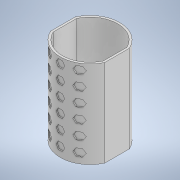
# Autodesk Inventor part: CanSat
Saved by Autodesk Inventor 2022 (Build 260153000, 153)
## iProperties
Created: 2022-01-26
Part Number: CanSat
Material: Generic
Document SubType Name: Modeling
Designer: jtgar
Density: 1 g/cm^3
Appearance: Default
Author: jtgar
Autodesk Inventor part; units mm, degrees
ref_plane "YZ Plane" through (0, 0, 0) normal (1, 0, 0) x (0, 1, 0)
ref_plane "XZ Plane" through (0, 0, 0) normal (0, 1, 0) x (-1, 0, 0)
ref_plane "XY Plane" through (0, 0, 0) normal (0, 0, 1) x (1, 0, 0)
sketch "Sketch1" plane through (0, 0, 0) normal (0, 1, 0) x (-1, 0, 0)
  circle A0 centre (0, 0) radius 28.5
  dimension "d0" = 57
  constraints: 1 centre point, 1 coincident
  measures "d0" diameter of A0
extrude "Extrusion1" add sketch "Sketch1" along normal blind 2.5
sketch "Sketch2" plane through (0, 2.5, 0) normal (0, 1, 0) x (1, 0, 0)
  circle A0 centre (0, 0) radius 27.5
  circle A1 centre (0, 0) radius 28.5
  dimension "d3" = 55
  dimension "d4" = 57
  constraints: 2 centre point, 2 coincident
  measures "d3" diameter of A0
  measures "d4" diameter of A1
sketch "Sketch3" plane through (0, 0, 0) normal (0, 0, 1) x (1, 0, 0)
  line L0 (-4.0696, 9.3373) -> (-2.0348, 12.8616)
  line L1 (-2.0348, 12.8616) -> (2.0348, 12.8616)
  line L2 (2.0348, 12.8616) -> (4.0696, 9.3373)
  line L3 (4.0696, 9.3373) -> (2.0348, 5.8129)
  line L4 (2.0348, 5.8129) -> (-2.0348, 5.8129)
  line L5 (-2.0348, 5.8129) -> (-4.0696, 9.3373)
  line L6 (4.0696, 9.3373) -> (2.0348, 12.8616)
  line L7 (2.0348, 12.8616) -> (-2.0348, 12.8616)
  line L8 (-2.0348, 12.8616) -> (-4.0696, 9.3373)
  line L9 (-4.0696, 9.3373) -> (-2.0348, 5.8129)
  line L10 (-2.0348, 5.8129) -> (2.0348, 5.8129)
  line L11 (2.0348, 5.8129) -> (4.0696, 9.3373)
  line L12 (4.0696, 9.3373) -> (2.0348, 12.8616)
  line L13 (2.0348, 12.8616) -> (-2.0348, 12.8616)
  line L14 (-2.0348, 12.8616) -> (-4.0696, 9.3373)
  line L15 (-4.0696, 9.3373) -> (-2.0348, 5.8129)
  line L16 (-2.0348, 5.8129) -> (2.0348, 5.8129)
  line L17 (2.0348, 5.8129) -> (4.0696, 9.3373)
  line L18 (-4.0696, 9.3373) -> (-2.0348, 12.8616)
  line L19 (-2.0348, 12.8616) -> (2.0348, 12.8616)
  line L20 (2.0348, 12.8616) -> (4.0696, 9.3373)
  line L21 (4.0696, 9.3373) -> (2.0348, 5.8129)
  line L22 (2.0348, 5.8129) -> (-2.0348, 5.8129)
  line L23 (-2.0348, 5.8129) -> (-4.0696, 9.3373)
  line L24 (28.5, 2.5) -> (-28.5, 2.5) projected
  line L25 (10.1843, 9.3373) -> (12.2172, 12.8582)
  line L26 (12.2172, 12.8582) -> (16.2828, 12.8582)
  line L27 (16.2828, 12.8582) -> (18.3157, 9.3373)
  line L28 (18.3157, 9.3373) -> (16.2828, 5.8163)
  line L29 (16.2828, 5.8163) -> (12.2172, 5.8163)
  line L30 (12.2172, 5.8163) -> (10.1843, 9.3373)
  line L31 (-18.3152, 9.3373) -> (-16.2826, 12.8579)
  line L32 (-16.2826, 12.8579) -> (-12.2174, 12.8579)
  line L33 (-12.2174, 12.8579) -> (-10.1848, 9.3373)
  line L34 (-10.1848, 9.3373) -> (-12.2174, 5.8166)
  line L35 (-12.2174, 5.8166) -> (-16.2826, 5.8166)
  line L36 (-16.2826, 5.8166) -> (-18.3152, 9.3373)
  line L37 (-4.0696, 23.012) -> (-2.0348, 19.4877)
  line L38 (-2.0348, 19.4877) -> (2.0348, 19.4877)
  line L39 (2.0348, 19.4877) -> (4.0696, 23.012)
  line L40 (4.0696, 23.012) -> (2.0348, 26.5364)
  line L41 (2.0348, 26.5364) -> (-2.0348, 26.5364)
  line L42 (-2.0348, 26.5364) -> (-4.0696, 23.012)
  line L43 (4.0696, 23.012) -> (2.0348, 19.4877)
  line L44 (2.0348, 19.4877) -> (-2.0348, 19.4877)
  line L45 (-2.0348, 19.4877) -> (-4.0696, 23.012)
  line L46 (-4.0696, 23.012) -> (-2.0348, 26.5364)
  line L47 (-2.0348, 26.5364) -> (2.0348, 26.5364)
  line L48 (2.0348, 26.5364) -> (4.0696, 23.012)
  line L49 (4.0696, 23.012) -> (2.0348, 19.4877)
  line L50 (2.0348, 19.4877) -> (-2.0348, 19.4877)
  line L51 (-2.0348, 19.4877) -> (-4.0696, 23.012)
  line L52 (-4.0696, 23.012) -> (-2.0348, 26.5364)
  line L53 (-2.0348, 26.5364) -> (2.0348, 26.5364)
  line L54 (2.0348, 26.5364) -> (4.0696, 23.012)
  line L55 (-4.0696, 23.012) -> (-2.0348, 19.4877)
  line L56 (-2.0348, 19.4877) -> (2.0348, 19.4877)
  line L57 (2.0348, 19.4877) -> (4.0696, 23.012)
  line L58 (4.0696, 23.012) -> (2.0348, 26.5364)
  line L59 (2.0348, 26.5364) -> (-2.0348, 26.5364)
  line L60 (-2.0348, 26.5364) -> (-4.0696, 23.012)
  line L61 (10.1843, 23.012) -> (12.2172, 19.491)
  line L62 (12.2172, 19.491) -> (16.2828, 19.491)
  line L63 (16.2828, 19.491) -> (18.3157, 23.012)
  line L64 (18.3157, 23.012) -> (16.2828, 26.533)
  line L65 (16.2828, 26.533) -> (12.2172, 26.533)
  line L66 (12.2172, 26.533) -> (10.1843, 23.012)
  line L67 (-18.3152, 23.012) -> (-16.2826, 19.4914)
  line L68 (-16.2826, 19.4914) -> (-12.2174, 19.4914)
  line L69 (-12.2174, 19.4914) -> (-10.1848, 23.012)
  line L70 (-10.1848, 23.012) -> (-12.2174, 26.5326)
  line L71 (-12.2174, 26.5326) -> (-16.2826, 26.5326)
  line L72 (-16.2826, 26.5326) -> (-18.3152, 23.012)
  line L73 (-4.0696, 50.362) -> (-2.0348, 46.8377)
  line L74 (-2.0348, 46.8377) -> (2.0348, 46.8377)
  line L75 (2.0348, 46.8377) -> (4.0696, 50.362)
  line L76 (4.0696, 50.362) -> (2.0348, 53.8864)
  line L77 (2.0348, 53.8864) -> (-2.0348, 53.8864)
  line L78 (-2.0348, 53.8864) -> (-4.0696, 50.362)
  line L79 (4.0696, 50.362) -> (2.0348, 46.8377)
  line L80 (2.0348, 46.8377) -> (-2.0348, 46.8377)
  line L81 (-2.0348, 46.8377) -> (-4.0696, 50.362)
  line L82 (-4.0696, 50.362) -> (-2.0348, 53.8864)
  line L83 (-2.0348, 53.8864) -> (2.0348, 53.8864)
  line L84 (2.0348, 53.8864) -> (4.0696, 50.362)
  line L85 (4.0696, 50.362) -> (2.0348, 46.8377)
  line L86 (2.0348, 46.8377) -> (-2.0348, 46.8377)
  line L87 (-2.0348, 46.8377) -> (-4.0696, 50.362)
  line L88 (-4.0696, 50.362) -> (-2.0348, 53.8864)
  line L89 (-2.0348, 53.8864) -> (2.0348, 53.8864)
  line L90 (2.0348, 53.8864) -> (4.0696, 50.362)
  line L91 (-4.0696, 50.362) -> (-2.0348, 46.8377)
  line L92 (-2.0348, 46.8377) -> (2.0348, 46.8377)
  line L93 (2.0348, 46.8377) -> (4.0696, 50.362)
  line L94 (4.0696, 50.362) -> (2.0348, 53.8864)
  line L95 (2.0348, 53.8864) -> (-2.0348, 53.8864)
  line L96 (-2.0348, 53.8864) -> (-4.0696, 50.362)
  line L97 (10.1843, 50.362) -> (12.2172, 46.841)
  line L98 (12.2172, 46.841) -> (16.2828, 46.841)
  line L99 (16.2828, 46.841) -> (18.3157, 50.362)
  line L100 (18.3157, 50.362) -> (16.2828, 53.883)
  line L101 (16.2828, 53.883) -> (12.2172, 53.883)
  line L102 (12.2172, 53.883) -> (10.1843, 50.362)
  line L103 (-18.3152, 50.362) -> (-16.2826, 46.8414)
  line L104 (-16.2826, 46.8414) -> (-12.2174, 46.8414)
  line L105 (-12.2174, 46.8414) -> (-10.1848, 50.362)
  line L106 (-10.1848, 50.362) -> (-12.2174, 53.8826)
  line L107 (-12.2174, 53.8826) -> (-16.2826, 53.8826)
  line L108 (-16.2826, 53.8826) -> (-18.3152, 50.362)
  line L109 (-2.0348, 33.1629) -> (2.0348, 33.1629)
  line L110 (-2.0348, 33.1629) -> (2.0348, 33.1629)
  line L111 (2.0348, 33.1629) -> (-2.0348, 33.1629)
  line L112 (2.0348, 33.1629) -> (-2.0348, 33.1629)
  line L113 (4.0696, 36.6873) -> (2.0348, 33.1629)
  line L114 (4.0696, 36.6873) -> (2.0348, 33.1629)
  line L115 (2.0348, 33.1629) -> (4.0696, 36.6873)
  line L116 (2.0348, 33.1629) -> (4.0696, 36.6873)
  line L117 (2.0348, 40.2116) -> (4.0696, 36.6873)
  line L118 (4.0696, 36.6873) -> (2.0348, 40.2116)
  line L119 (4.0696, 36.6873) -> (2.0348, 40.2116)
  line L120 (2.0348, 40.2116) -> (4.0696, 36.6873)
  line L121 (2.0348, 40.2116) -> (-2.0348, 40.2116)
  line L122 (2.0348, 40.2116) -> (-2.0348, 40.2116)
  line L123 (-2.0348, 40.2116) -> (2.0348, 40.2116)
  line L124 (-2.0348, 40.2116) -> (2.0348, 40.2116)
  line L125 (10.1843, 36.6873) -> (12.2172, 40.2082)
  line L126 (12.2172, 33.1663) -> (10.1843, 36.6873)
  line L127 (12.2172, 40.2082) -> (16.2828, 40.2082)
  line L128 (16.2828, 33.1663) -> (12.2172, 33.1663)
  line L129 (18.3157, 36.6873) -> (16.2828, 33.1663)
  line L130 (16.2828, 40.2082) -> (18.3157, 36.6873)
  line L131 (-4.0696, 36.6873) -> (-2.0348, 40.2116)
  line L132 (-2.0348, 33.1629) -> (-4.0696, 36.6873)
  line L133 (-2.0348, 40.2116) -> (-4.0696, 36.6873)
  line L134 (-4.0696, 36.6873) -> (-2.0348, 33.1629)
  line L135 (-2.0348, 40.2116) -> (-4.0696, 36.6873)
  line L136 (-4.0696, 36.6873) -> (-2.0348, 33.1629)
  line L137 (-4.0696, 36.6873) -> (-2.0348, 40.2116)
  line L138 (-2.0348, 33.1629) -> (-4.0696, 36.6873)
  line L139 (-12.2174, 40.2079) -> (-10.1848, 36.6873)
  line L140 (-16.2826, 40.2079) -> (-12.2174, 40.2079)
  line L141 (-12.2174, 33.1666) -> (-16.2826, 33.1666)
  line L142 (-18.3152, 36.6873) -> (-16.2826, 40.2079)
  line L143 (-16.2826, 33.1666) -> (-18.3152, 36.6873)
  line L144 (-10.1848, 36.6873) -> (-12.2174, 33.1666)
  line L145 (-4.0696, 105.0625) -> (-2.0348, 101.5381)
  line L146 (-2.0348, 101.5381) -> (2.0348, 101.5381)
  line L147 (2.0348, 101.5381) -> (4.0696, 105.0625)
  line L148 (4.0696, 105.0625) -> (2.0348, 108.5868)
  line L149 (2.0348, 108.5868) -> (-2.0348, 108.5868)
  line L150 (-2.0348, 108.5868) -> (-4.0696, 105.0625)
  line L151 (4.0696, 105.0625) -> (2.0348, 101.5381)
  line L152 (2.0348, 101.5381) -> (-2.0348, 101.5381)
  line L153 (-2.0348, 101.5381) -> (-4.0696, 105.0625)
  line L154 (-4.0696, 105.0625) -> (-2.0348, 108.5868)
  line L155 (-2.0348, 108.5868) -> (2.0348, 108.5868)
  line L156 (2.0348, 108.5868) -> (4.0696, 105.0625)
  line L157 (4.0696, 105.0625) -> (2.0348, 101.5381)
  line L158 (2.0348, 101.5381) -> (-2.0348, 101.5381)
  line L159 (-2.0348, 101.5381) -> (-4.0696, 105.0625)
  line L160 (-4.0696, 105.0625) -> (-2.0348, 108.5868)
  line L161 (-2.0348, 108.5868) -> (2.0348, 108.5868)
  line L162 (2.0348, 108.5868) -> (4.0696, 105.0625)
  line L163 (-4.0696, 105.0625) -> (-2.0348, 101.5381)
  line L164 (-2.0348, 101.5381) -> (2.0348, 101.5381)
  line L165 (2.0348, 101.5381) -> (4.0696, 105.0625)
  line L166 (4.0696, 105.0625) -> (2.0348, 108.5868)
  line L167 (2.0348, 108.5868) -> (-2.0348, 108.5868)
  line L168 (-2.0348, 108.5868) -> (-4.0696, 105.0625)
  line L169 (10.1843, 105.0625) -> (12.2172, 101.5415)
  line L170 (12.2172, 101.5415) -> (16.2828, 101.5415)
  line L171 (16.2828, 101.5415) -> (18.3157, 105.0625)
  line L172 (18.3157, 105.0625) -> (16.2828, 108.5835)
  line L173 (16.2828, 108.5835) -> (12.2172, 108.5835)
  line L174 (12.2172, 108.5835) -> (10.1843, 105.0625)
  line L175 (-18.3152, 105.0625) -> (-16.2826, 101.5419)
  line L176 (-16.2826, 101.5419) -> (-12.2174, 101.5419)
  line L177 (-12.2174, 101.5419) -> (-10.1848, 105.0625)
  line L178 (-10.1848, 105.0625) -> (-12.2174, 108.5831)
  line L179 (-12.2174, 108.5831) -> (-16.2826, 108.5831)
  line L180 (-16.2826, 108.5831) -> (-18.3152, 105.0625)
  line L181 (-2.0348, 87.8633) -> (2.0348, 87.8633)
  line L182 (-2.0348, 87.8633) -> (2.0348, 87.8633)
  line L183 (2.0348, 87.8633) -> (-2.0348, 87.8633)
  line L184 (2.0348, 87.8633) -> (-2.0348, 87.8633)
  line L185 (4.0696, 91.3877) -> (2.0348, 87.8633)
  line L186 (4.0696, 91.3877) -> (2.0348, 87.8633)
  line L187 (2.0348, 87.8633) -> (4.0696, 91.3877)
  line L188 (2.0348, 87.8633) -> (4.0696, 91.3877)
  line L189 (2.0348, 94.9121) -> (4.0696, 91.3877)
  line L190 (4.0696, 91.3877) -> (2.0348, 94.9121)
  line L191 (4.0696, 91.3877) -> (2.0348, 94.9121)
  line L192 (2.0348, 94.9121) -> (4.0696, 91.3877)
  line L193 (2.0348, 94.9121) -> (-2.0348, 94.9121)
  line L194 (2.0348, 94.9121) -> (-2.0348, 94.9121)
  line L195 (-2.0348, 94.9121) -> (2.0348, 94.9121)
  line L196 (-2.0348, 94.9121) -> (2.0348, 94.9121)
  line L197 (10.1843, 91.3877) -> (12.2172, 94.9087)
  line L198 (12.2172, 87.8667) -> (10.1843, 91.3877)
  line L199 (12.2172, 94.9087) -> (16.2828, 94.9087)
  line L200 (16.2828, 87.8667) -> (12.2172, 87.8667)
  line L201 (18.3157, 91.3877) -> (16.2828, 87.8667)
  line L202 (16.2828, 94.9087) -> (18.3157, 91.3877)
  line L203 (-4.0696, 91.3877) -> (-2.0348, 94.9121)
  line L204 (-2.0348, 87.8633) -> (-4.0696, 91.3877)
  line L205 (-2.0348, 94.9121) -> (-4.0696, 91.3877)
  line L206 (-4.0696, 91.3877) -> (-2.0348, 87.8633)
  line L207 (-2.0348, 94.9121) -> (-4.0696, 91.3877)
  line L208 (-4.0696, 91.3877) -> (-2.0348, 87.8633)
  line L209 (-4.0696, 91.3877) -> (-2.0348, 94.9121)
  line L210 (-2.0348, 87.8633) -> (-4.0696, 91.3877)
  line L211 (-12.2174, 94.9083) -> (-10.1848, 91.3877)
  line L212 (-16.2826, 94.9083) -> (-12.2174, 94.9083)
  line L213 (-12.2174, 87.8671) -> (-16.2826, 87.8671)
  line L214 (-18.3152, 91.3877) -> (-16.2826, 94.9083)
  line L215 (-16.2826, 87.8671) -> (-18.3152, 91.3877)
  line L216 (-10.1848, 91.3877) -> (-12.2174, 87.8671)
  line L217 (-2.0348, 67.5621) -> (2.0348, 67.5621)
  line L218 (-2.0348, 67.5621) -> (2.0348, 67.5621)
  line L219 (2.0348, 67.5621) -> (4.0696, 64.0377)
  line L220 (2.0348, 67.5621) -> (4.0696, 64.0377)
  line L221 (10.1843, 77.7125) -> (12.2172, 74.1915)
  line L222 (2.0348, 67.5621) -> (-2.0348, 67.5621)
  line L223 (2.0348, 67.5621) -> (-2.0348, 67.5621)
  line L224 (-4.0696, 64.0377) -> (-2.0348, 67.5621)
  line L225 (-2.0348, 67.5621) -> (-4.0696, 64.0377)
  line L226 (-2.0348, 67.5621) -> (-4.0696, 64.0377)
  line L227 (4.0696, 64.0377) -> (2.0348, 67.5621)
  line L228 (4.0696, 64.0377) -> (2.0348, 67.5621)
  line L229 (2.0348, 60.5133) -> (-2.0348, 60.5133)
  line L230 (4.0696, 64.0377) -> (2.0348, 60.5133)
  line L231 (2.0348, 60.5133) -> (4.0696, 64.0377)
  line L232 (10.1843, 64.0377) -> (12.2172, 67.5587)
  line L233 (12.2172, 67.5587) -> (16.2828, 67.5587)
  line L234 (12.2172, 74.1915) -> (16.2828, 74.1915)
  line L235 (16.2828, 60.5167) -> (12.2172, 60.5167)
  line L236 (12.2172, 81.2335) -> (10.1843, 77.7125)
  line L237 (-2.0348, 60.5133) -> (-4.0696, 64.0377)
  line L238 (-2.0348, 60.5133) -> (2.0348, 60.5133)
  line L239 (-4.0696, 64.0377) -> (-2.0348, 60.5133)
  line L240 (18.3157, 64.0377) -> (16.2828, 60.5167)
  line L241 (16.2828, 67.5587) -> (18.3157, 64.0377)
  line L242 (-4.0696, 64.0377) -> (-2.0348, 67.5621)
  line L243 (-4.0696, 64.0377) -> (-2.0348, 60.5133)
  line L244 (-2.0348, 60.5133) -> (2.0348, 60.5133)
  line L245 (2.0348, 60.5133) -> (4.0696, 64.0377)
  line L246 (2.0348, 60.5133) -> (-2.0348, 60.5133)
  line L247 (-2.0348, 60.5133) -> (-4.0696, 64.0377)
  line L248 (4.0696, 64.0377) -> (2.0348, 60.5133)
  line L249 (16.2828, 74.1915) -> (18.3157, 77.7125)
  line L250 (16.2828, 81.2335) -> (12.2172, 81.2335)
  line L251 (18.3157, 77.7125) -> (16.2828, 81.2335)
  line L252 (12.2172, 60.5167) -> (10.1843, 64.0377)
  line L253 (2.0348, 81.2368) -> (-2.0348, 81.2368)
  line L254 (2.0348, 81.2368) -> (-2.0348, 81.2368)
  line L255 (-2.0348, 81.2368) -> (2.0348, 81.2368)
  line L256 (-2.0348, 81.2368) -> (2.0348, 81.2368)
  line L257 (-4.0696, 77.7125) -> (-2.0348, 81.2368)
  line L258 (-4.0696, 77.7125) -> (-2.0348, 81.2368)
  line L259 (-2.0348, 81.2368) -> (-4.0696, 77.7125)
  line L260 (-2.0348, 81.2368) -> (-4.0696, 77.7125)
  line L261 (-2.0348, 74.1881) -> (-4.0696, 77.7125)
  line L262 (-2.0348, 74.1881) -> (-4.0696, 77.7125)
  line L263 (-4.0696, 77.7125) -> (-2.0348, 74.1881)
  line L264 (-4.0696, 77.7125) -> (-2.0348, 74.1881)
  line L265 (-2.0348, 74.1881) -> (2.0348, 74.1881)
  line L266 (-2.0348, 74.1881) -> (2.0348, 74.1881)
  line L267 (2.0348, 74.1881) -> (-2.0348, 74.1881)
  line L268 (2.0348, 74.1881) -> (-2.0348, 74.1881)
  line L269 (4.0696, 77.7125) -> (2.0348, 81.2368)
  line L270 (4.0696, 77.7125) -> (2.0348, 81.2368)
  line L271 (4.0696, 77.7125) -> (2.0348, 74.1881)
  line L272 (4.0696, 77.7125) -> (2.0348, 74.1881)
  line L273 (2.0348, 81.2368) -> (4.0696, 77.7125)
  line L274 (2.0348, 74.1881) -> (4.0696, 77.7125)
  line L275 (2.0348, 74.1881) -> (4.0696, 77.7125)
  line L276 (2.0348, 81.2368) -> (4.0696, 77.7125)
  line L277 (-18.3152, 64.0377) -> (-16.2826, 67.5583)
  line L278 (-16.2826, 67.5583) -> (-12.2174, 67.5583)
  line L279 (-12.2174, 67.5583) -> (-10.1848, 64.0377)
  line L280 (-10.1848, 64.0377) -> (-12.2174, 60.5171)
  line L281 (-12.2174, 60.5171) -> (-16.2826, 60.5171)
  line L282 (-16.2826, 60.5171) -> (-18.3152, 64.0377)
  line L283 (-16.2826, 74.1919) -> (-12.2174, 74.1919)
  line L284 (-12.2174, 74.1919) -> (-10.1848, 77.7125)
  line L285 (-12.2174, 81.2331) -> (-16.2826, 81.2331)
  line L286 (-10.1848, 77.7125) -> (-12.2174, 81.2331)
  line L287 (-18.3152, 77.7125) -> (-16.2826, 74.1919)
  line L288 (-16.2826, 81.2331) -> (-18.3152, 77.7125)
  point P0 (0, 0)
  point P1 (0, 9.3373)
  point P2 (14.25, 9.3373)
  point P3 (-14.25, 9.3373)
  point P4 (0, 23.012)
  point P5 (14.25, 23.012)
  point P6 (-14.25, 23.012)
  point P7 (0, 50.362)
  point P8 (14.25, 50.362)
  point P9 (-14.25, 50.362)
  point P10 (0, 36.6873)
  point P11 (14.25, 36.6873)
  point P12 (-14.25, 36.6873)
  point P13 (0, 105.0625)
  point P14 (0, 61.7829)
  point P15 (14.25, 62.2333)
  point P16 (-14.25, 62.2333)
  point P17 (14.25, 105.0625)
  point P18 (-14.25, 105.0625)
  point P19 (0, 91.3877)
  point P20 (14.25, 91.3877)
  point P21 (-14.25, 91.3877)
  point P22 (0, 64.0377)
  point P23 (14.25, 64.0377)
  point P24 (14.25, 77.7125)
  point P25 (0, 77.7125)
  point P26 (-14.25, 64.0377)
  point P27 (-14.25, 77.7125)
  constraints: 576 end point, 39 other
extrude "Extrusion2" add sketch "Sketch2" along normal blind 110
extrude "Extrusion3" cut sketch "Sketch3" along normal mid plane 110
sketch "Sketch4" plane through (0, 0, 0) normal (0, 0, 1) x (1, 0, 0)
  line L0 (27.5, 2.5) -> (-27.5, 2.5) projected
  line L1 (0, 2.5) -> (0, 83.5)
  line L2 (0, 83.5) -> (36.3066, 83.5)
  line L3 (36.3066, 83.5) -> (-38.1536, 83.5)
  line L4 (-38.1536, 83.5) -> (-38.1536, 115.4142)
  line L5 (-38.1536, 115.4142) -> (36.3066, 115.4142)
  line L6 (36.3066, 115.4142) -> (36.3066, 83.5)
  point P0 (0, 0)
  dimension "d13" = 81
  constraints: 12 end point, 3 perpendicular, 1 horizontal, 1 midpoint, 1 point on line, 1 vertical
  measures "d13" distance of L1.start L1.end
extrude "Extrusion4" cut sketch "Sketch4" along normal mid plane 110
sketch "Sketch5" plane through (0, 83.5, 0) normal (0, 1, 0) x (1, 0, 0)
  line L0 (-26, 0) -> (-26, -24.5085)
  line L1 (-26, -23.9178) -> (-26, 18.195)
  line L2 (-26, 18.195) -> (-32.2303, 18.195)
  line L3 (-32.2303, 18.195) -> (-32.2303, -24.5085)
  line L4 (-32.2303, -24.5085) -> (-26, -24.5085)
  line L5 (0, 5.9637) -> (0, -3.1567)
  line L6 (26, -24.5085) -> (26, 18.195)
  line L7 (26, 18.195) -> (32.2303, 18.195)
  line L8 (32.2303, 18.195) -> (32.2303, -24.5085)
  line L9 (32.2303, -24.5085) -> (26, -24.5085)
  point P0 (0, 0)
  point P1 (26, -23.9178)
  constraints: 20 end point, 5 symmetric about line, 4 point on line, 2 perpendicular, 2 vertical, 1 parallel
extrude "Extrusion5" cut sketch "Sketch5" against normal through all
sketch "Sketch6" plane through (0, 2.5, 0) normal (0, 1, 0) x (1, 0, 0)
  arc A0 (26, 11.6726) -> (-26, 11.6726) centre (0, 0) ccw projected
  line L0 (-26, 11.6726) -> (-24.8998, 11.6726)
  arc A1 (26, 8.9582) -> (-26, 8.9582) centre (0, 0) ccw projected
  circle A2 centre (0, 0) radius 26.5
  line L1 (-26, 8.9582) -> (-26, -8.9582) projected
  line L2 (-26, 0) -> (-24, 0)
  line L3 (-24, 0) -> (-24, 11.2361)
  line L4 (-24, 0) -> (-24, -11.2361)
  line L5 (26, 11.6726) -> (26, -11.6726) projected
  line L6 (26, 0) -> (24, 0)
  line L7 (24, 0) -> (24, 11.2361)
  line L8 (24, 0) -> (24, -11.2361)
  arc A3 (-26, -8.9582) -> (26, -8.9582) centre (0, 0) ccw projected
  line L9 (-26, -8.9582) -> (-26, -5.1235)
  line L10 (26, -8.9582) -> (26, -5.1235)
  dimension "d18" = 53
  dimension "d19" = 2
  dimension "d20" = 2
  constraints: 18 end point, 7 point on circle, 6 point on line, 2 horizontal, 2 midpoint, 2 perpendicular, 1 centre point, 1 coincident
  measures "d18" diameter of A2
  measures "d19" distance of L2.start L2.end
  measures "d20" distance of L6.start L6.end
extrude "Extrusion6" add sketch "Sketch6" along normal blind 81 contours L5 A2 L1 A1 | L5 L6 L7 A2 | L5 A2 L8 L6 | A2 L3 L2 L1 | L5 A3 L1 A2 | L1 L2 L4 A2
body "Solid1"
